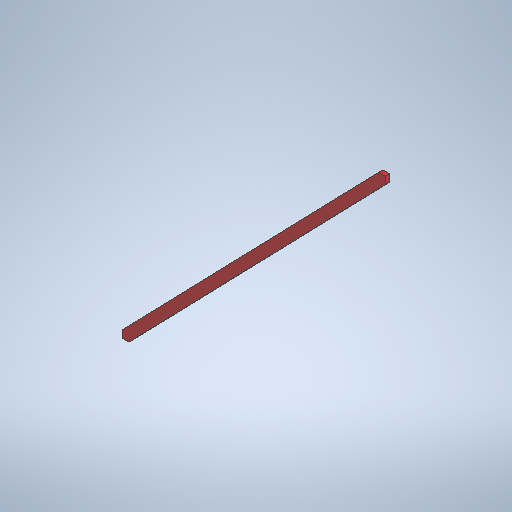
# Autodesk Inventor part: s88x2x4
Saved by Autodesk Inventor 2025.1 (Build 291241020, 241B)
## iProperties
Created: 2024-09-19
Part Number: s88x2x4
Material: Generic
Document SubType Name: Modeling
Designer: User
Density: 1 g/cm^3
Appearance: Default
Author: User
Autodesk Inventor part; units mm, degrees
ref_plane "YZ Plane" through (0, 0, 0) normal (1, 0, 0) x (0, 1, 0)
ref_plane "XZ Plane" through (0, 0, 0) normal (0, 1, 0) x (-1, 0, 0)
ref_plane "XY Plane" through (0, 0, 0) normal (0, 0, 1) x (1, 0, 0)
ref_plane "Work Plane1" through (0, 0, 1200.15) normal (0, 0, 1) x (0, 1, 0)
sketch "Sketch1" plane through (0, 0, 1200.15) normal (0, 0, 1) x (0, 1, 0)
  line L0 (0, -2400.3) -> (2438.4, -2400.3) projected
  line L1 (2438.4, 0) -> (2438.4, -2438.4) projected
  line L2 (0, 0) -> (0, -3657.6) projected
  line L3 (0, -38.1) -> (2438.4, -38.1) projected
  line L4 (63.8837, -38.1) -> (2438.4, -2338.4126)
  line L5 (2438.4, -2338.4126) -> (2438.4, -2400.3)
  line L6 (2438.4, -2400.3) -> (2374.5163, -2400.3)
  line L7 (2374.5163, -2400.3) -> (0, -99.9874)
  line L8 (0, -99.9874) -> (0, -38.1)
  line L9 (0, -38.1) -> (63.8837, -38.1)
  constraints: 12 end point, 4 point on line, 3 collinear, 1 parallel, 2 other
extrude "Extrusion1" add sketch "Sketch1" against normal blind 38.1 contours L7 L2 L3 L4 L1 L0
body "Solid1"
